Autodesk Fusion 360 part; units mm, degrees
(part 4 of 7)
  line L870 (66.9243, -68.9138) -> (66.9958, -68.9472)
  line L871 (66.9958, -68.9472) -> (67.1016, -68.8548)
  line L872 (67.1016, -68.8548) -> (67.2059, -68.7609)
  line L873 (67.2059, -68.7609) -> (67.3089, -68.6653)
  line L874 (67.3089, -68.6653) -> (67.2831, -68.5907)
  line L875 (67.2831, -68.5907) -> (67.256, -68.5172)
  line L876 (67.256, -68.5172) -> (67.2276, -68.4449)
  line L877 (67.2276, -68.4449) -> (67.1977, -68.3739)
  line L878 (67.1977, -68.3739) -> (67.1663, -68.3041)
  line L879 (67.1663, -68.3041) -> (67.1335, -68.2357)
  line L880 (67.1335, -68.2357) -> (67.099, -68.1688)
  line L881 (67.099, -68.1688) -> (67.0628, -68.1036)
  line L882 (67.0628, -68.1036) -> (67.0248, -68.04)
  line L883 (67.0248, -68.04) -> (66.9847, -67.9785)
  line L884 (66.9847, -67.9785) -> (66.942, -67.9195)
  line L885 (66.942, -67.9195) -> (66.8957, -67.8642)
  line L886 (66.8957, -67.8642) -> (66.5795, -67.5479)
  line L887 (66.5795, -67.5479) -> (66.7269, -67.3967)
  line L888 (66.7269, -67.3967) -> (66.8702, -67.2417)
  line L889 (66.8702, -67.2417) -> (67.0094, -67.0829)
  line L890 (67.0094, -67.0829) -> (67.1444, -66.9206)
  line L891 (67.1444, -66.9206) -> (67.492, -67.2019)
  line L892 (67.492, -67.2019) -> (67.5519, -67.2422)
  line L893 (67.5519, -67.2422) -> (67.615, -67.2785)
  line L894 (67.615, -67.2785) -> (67.6804, -67.3119)
  line L895 (67.6804, -67.3119) -> (67.7475, -67.3431)
  line L896 (67.7475, -67.3431) -> (67.8162, -67.3723)
  line L897 (67.8162, -67.3723) -> (67.8864, -67.3996)
  line L898 (67.8864, -67.3996) -> (67.9578, -67.4251)
  line L899 (67.9578, -67.4251) -> (68.0305, -67.449)
  line L900 (68.0305, -67.449) -> (68.1043, -67.4713)
  line L901 (68.1043, -67.4713) -> (68.1791, -67.492)
  line L902 (68.1791, -67.492) -> (68.255, -67.5113)
  line L903 (68.255, -67.5113) -> (68.3319, -67.5291)
  line L904 (68.3319, -67.5291) -> (68.4162, -67.4167)
  line L905 (68.4162, -67.4167) -> (68.4987, -67.3031)
  line L906 (68.4987, -67.3031) -> (68.5795, -67.1883)
  line L907 (68.5795, -67.1883) -> (68.5389, -67.1207)
  line L908 (68.5389, -67.1207) -> (68.4971, -67.0544)
  line L909 (68.4971, -67.0544) -> (68.4542, -66.9896)
  line L910 (68.4542, -66.9896) -> (68.4102, -66.9263)
  line L911 (68.4102, -66.9263) -> (68.365, -66.8646)
  line L912 (68.365, -66.8646) -> (68.3187, -66.8046)
  line L913 (68.3187, -66.8046) -> (68.271, -66.7463)
  line L914 (68.271, -66.7463) -> (68.2221, -66.6899)
  line L915 (68.2221, -66.6899) -> (68.1717, -66.6357)
  line L916 (68.1717, -66.6357) -> (68.1196, -66.5839)
  line L917 (68.1196, -66.5839) -> (68.0657, -66.535)
  line L918 (68.0657, -66.535) -> (68.0088, -66.4906)
  line L919 (68.0088, -66.4906) -> (67.6338, -66.2469)
  line L920 (67.6338, -66.2469) -> (67.7465, -66.0684)
  line L921 (67.7465, -66.0684) -> (67.8545, -65.8869)
  line L922 (67.8545, -65.8869) -> (67.9576, -65.7027)
  line L923 (67.9576, -65.7027) -> (68.0559, -65.5158)
  line L924 (68.0559, -65.5158) -> (68.4544, -65.7187)
  line L925 (68.4544, -65.7187) -> (68.5214, -65.7458)
  line L926 (68.5214, -65.7458) -> (68.5907, -65.7681)
  line L927 (68.5907, -65.7681) -> (68.6615, -65.7872)
  line L928 (68.6615, -65.7872) -> (68.7337, -65.8038)
  line L929 (68.7337, -65.8038) -> (68.807, -65.818)
  line L930 (68.807, -65.818) -> (68.8813, -65.8301)
  line L931 (68.8813, -65.8301) -> (68.9564, -65.8402)
  line L932 (68.9564, -65.8402) -> (69.0325, -65.8485)
  line L933 (69.0325, -65.8485) -> (69.1093, -65.855)
  line L934 (69.1093, -65.855) -> (69.1869, -65.8597)
  line L935 (69.1869, -65.8597) -> (69.2651, -65.8627)
  line L936 (69.2651, -65.8627) -> (69.344, -65.8642)
  line L937 (69.344, -65.8642) -> (69.4031, -65.7368)
  line L938 (69.4031, -65.7368) -> (69.4602, -65.6085)
  line L939 (69.4602, -65.6085) -> (69.5154, -65.4793)
  line L940 (69.5154, -65.4793) -> (69.4615, -65.4216)
  line L941 (69.4615, -65.4216) -> (69.4069, -65.3655)
  line L942 (69.4069, -65.3655) -> (69.3515, -65.3111)
  line L943 (69.3515, -65.3111) -> (69.2952, -65.2583)
  line L944 (69.2952, -65.2583) -> (69.2382, -65.2073)
  line L945 (69.2382, -65.2073) -> (69.1804, -65.1582)
  line L946 (69.1804, -65.1582) -> (69.1217, -65.1111)
  line L947 (69.1217, -65.1111) -> (69.0621, -65.0662)
  line L948 (69.0621, -65.0662) -> (69.0015, -65.0236)
  line L949 (69.0015, -65.0236) -> (68.9399, -64.9838)
  line L950 (68.9399, -64.9838) -> (68.8769, -64.9472)
  line L951 (68.8769, -64.9472) -> (68.812, -64.9156)
  line L952 (68.812, -64.9156) -> (68.3946, -64.7551)
  line L953 (68.3946, -64.7551) -> (68.4677, -64.5571)
  line L954 (68.4677, -64.5571) -> (68.5356, -64.3572)
  line L955 (68.5356, -64.3572) -> (68.5982, -64.1555)
  line L956 (68.5982, -64.1555) -> (68.6554, -63.9523)
  line L957 (68.6554, -63.9523) -> (69.0875, -64.0679)
  line L958 (69.0875, -64.0679) -> (69.1585, -64.0804)
  line L959 (69.1585, -64.0804) -> (69.231, -64.0878)
  line L960 (69.231, -64.0878) -> (69.3043, -64.0918)
  line L961 (69.3043, -64.0918) -> (69.3783, -64.093)
  line L962 (69.3783, -64.093) -> (69.4529, -64.0917)
  line L963 (69.4529, -64.0917) -> (69.5281, -64.0881)
  line L964 (69.5281, -64.0881) -> (69.6038, -64.0824)
  line L965 (69.6038, -64.0824) -> (69.6798, -64.0746)
  line L966 (69.6798, -64.0746) -> (69.7563, -64.065)
  line L967 (69.7563, -64.065) -> (69.8332, -64.0535)
  line L968 (69.8332, -64.0535) -> (69.9104, -64.0402)
  line L969 (69.9104, -64.0402) -> (69.9878, -64.0252)
  line L970 (69.9878, -64.0252) -> (70.0191, -63.8883)
  line L971 (70.0191, -63.8883) -> (70.0483, -63.7509)
  line L972 (70.0483, -63.7509) -> (70.0754, -63.6131)
  line L973 (70.0754, -63.6131) -> (70.0107, -63.5679)
  line L974 (70.0107, -63.5679) -> (69.9456, -63.5244)
  line L975 (69.9456, -63.5244) -> (69.8801, -63.4826)
  line L976 (69.8801, -63.4826) -> (69.8142, -63.4427)
  line L977 (69.8142, -63.4427) -> (69.7478, -63.4047)
  line L978 (69.7478, -63.4047) -> (69.681, -63.3687)
  line L979 (69.681, -63.3687) -> (69.6138, -63.3348)
  line L980 (69.6138, -63.3348) -> (69.5462, -63.3033)
  line L981 (69.5462, -63.3033) -> (69.4781, -63.2742)
  line L982 (69.4781, -63.2742) -> (69.4095, -63.2481)
  line L983 (69.4095, -63.2481) -> (69.3403, -63.2254)
  line L984 (69.3403, -63.2254) -> (69.2703, -63.2079)
  line L985 (69.2703, -63.2079) -> (68.8286, -63.1378)
  line L986 (68.8286, -63.1378) -> (68.8589, -62.9289)
  line L987 (68.8589, -62.9289) -> (68.8837, -62.7192)
  line L988 (68.8837, -62.7192) -> (68.903, -62.509)
  line L989 (68.903, -62.509) -> (68.9168, -62.2983)
  circle A0 centre (60.9176, -61.8819) radius 2
extrude "Extrude1''" add sketch "Sketch1 (3)" along normal blind 2 separate body makes body 5 in component "CT idler 2"
ref_plane "WorkPlane2" through (0, 0, 41.2) normal (0, 0, 1) x (1, 0, 0) in component "CT idler 2"
sketch "Sketch2 (2)" plane through (0, 0, 41.2) normal (0, 0, 1) x (1, 0, 0) in component "CT idler 2"
  line L0 (63.97, -62.3626) -> (64.2593, -62.4081)
  line L1 (64.2593, -62.4081) -> (64.3399, -62.409)
  line L2 (64.3399, -62.409) -> (64.422, -62.3998)
  line L3 (64.422, -62.3998) -> (64.5049, -62.3837)
  line L4 (64.5049, -62.3837) -> (64.5883, -62.3617)
  line L5 (64.5883, -62.3617) -> (64.6722, -62.3342)
  line L6 (64.6722, -62.3342) -> (64.7562, -62.3017)
  line L7 (64.7562, -62.3017) -> (64.8402, -62.2644)
  line L8 (64.8402, -62.2644) -> (64.9242, -62.2224)
  line L9 (64.9242, -62.2224) -> (65.0078, -62.1758)
  line L10 (65.0078, -62.1758) -> (65.091, -62.1248)
  line L11 (65.091, -62.1248) -> (65.1737, -62.0695)
  line L12 (65.1737, -62.0695) -> (65.2557, -62.0099)
  line L13 (65.2557, -62.0099) -> (65.2574, -61.9246)
  line L14 (65.2574, -61.9246) -> (65.2574, -61.8393)
  line L15 (65.2574, -61.8393) -> (65.2557, -61.754)
  line L16 (65.2557, -61.754) -> (65.1737, -61.6944)
  line L17 (65.1737, -61.6944) -> (65.091, -61.6391)
  line L18 (65.091, -61.6391) -> (65.0078, -61.5881)
  line L19 (65.0078, -61.5881) -> (64.9242, -61.5415)
  line L20 (64.9242, -61.5415) -> (64.8402, -61.4995)
  line L21 (64.8402, -61.4995) -> (64.7562, -61.4621)
  line L22 (64.7562, -61.4621) -> (64.6722, -61.4296)
  line L23 (64.6722, -61.4296) -> (64.5883, -61.4022)
  line L24 (64.5883, -61.4022) -> (64.5049, -61.3801)
  line L25 (64.5049, -61.3801) -> (64.422, -61.364)
  line L26 (64.422, -61.364) -> (64.3399, -61.3549)
  line L27 (64.3399, -61.3549) -> (64.2593, -61.3557)
  line L28 (64.2593, -61.3557) -> (63.97, -61.4013)
  line L29 (63.97, -61.4013) -> (63.9404, -61.2408)
  line L30 (63.9404, -61.2408) -> (63.9023, -61.0822)
  line L31 (63.9023, -61.0822) -> (63.856, -60.9257)
  line L32 (63.856, -60.9257) -> (63.8014, -60.772)
  line L33 (63.8014, -60.772) -> (64.0747, -60.6668)
  line L34 (64.0747, -60.6668) -> (64.145, -60.6272)
  line L35 (64.145, -60.6272) -> (64.2114, -60.5783)
  line L36 (64.2114, -60.5783) -> (64.2752, -60.5229)
  line L37 (64.2752, -60.5229) -> (64.3364, -60.4621)
  line L38 (64.3364, -60.4621) -> (64.3953, -60.3964)
  line L39 (64.3953, -60.3964) -> (64.4518, -60.3262)
  line L40 (64.4518, -60.3262) -> (64.5059, -60.2518)
  line L41 (64.5059, -60.2518) -> (64.5576, -60.1735)
  line L42 (64.5576, -60.1735) -> (64.6068, -60.0913)
  line L43 (64.6068, -60.0913) -> (64.6534, -60.0056)
  line L44 (64.6534, -60.0056) -> (64.6973, -59.9163)
  line L45 (64.6973, -59.9163) -> (64.7385, -59.8237)
  line L46 (64.7385, -59.8237) -> (64.6973, -59.749)
  line L47 (64.6973, -59.749) -> (64.6547, -59.6751)
  line L48 (64.6547, -59.6751) -> (64.6106, -59.6021)
  line L49 (64.6106, -59.6021) -> (64.5098, -59.5915)
  line L50 (64.5098, -59.5915) -> (64.4105, -59.5849)
  line L51 (64.4105, -59.5849) -> (64.3129, -59.5823)
  line L52 (64.3129, -59.5823) -> (64.2172, -59.5839)
  line L53 (64.2172, -59.5839) -> (64.1235, -59.5894)
  line L54 (64.1235, -59.5894) -> (64.032, -59.5991)
  line L55 (64.032, -59.5991) -> (63.943, -59.6129)
  line L56 (63.943, -59.6129) -> (63.8567, -59.6311)
  line L57 (63.8567, -59.6311) -> (63.7734, -59.6537)
  line L58 (63.7734, -59.6537) -> (63.6935, -59.6812)
  line L59 (63.6935, -59.6812) -> (63.6179, -59.7143)
  line L60 (63.6179, -59.7143) -> (63.5485, -59.7554)
  line L61 (63.5485, -59.7554) -> (63.3208, -59.9395)
  line L62 (63.3208, -59.9395) -> (63.2149, -59.8153)
  line L63 (63.2149, -59.8153) -> (63.1026, -59.697)
  line L64 (63.1026, -59.697) -> (62.9842, -59.5847)
  line L65 (62.9842, -59.5847) -> (62.8601, -59.4788)
  line L66 (62.8601, -59.4788) -> (63.0442, -59.251)
  line L67 (63.0442, -59.251) -> (63.0852, -59.1816)
  line L68 (63.0852, -59.1816) -> (63.1183, -59.106)
  line L69 (63.1183, -59.106) -> (63.1458, -59.0262)
  line L70 (63.1458, -59.0262) -> (63.1685, -58.9429)
  line L71 (63.1685, -58.9429) -> (63.1866, -58.8566)
  line L72 (63.1866, -58.8566) -> (63.2005, -58.7675)
  line L73 (63.2005, -58.7675) -> (63.2101, -58.6761)
  line L74 (63.2101, -58.6761) -> (63.2157, -58.5824)
  line L75 (63.2157, -58.5824) -> (63.2172, -58.4867)
  line L76 (63.2172, -58.4867) -> (63.2147, -58.3891)
  line L77 (63.2147, -58.3891) -> (63.2081, -58.2898)
  line L78 (63.2081, -58.2898) -> (63.1975, -58.189)
  line L79 (63.1975, -58.189) -> (63.1245, -58.1449)
  line L80 (63.1245, -58.1449) -> (63.0506, -58.1022)
  line L81 (63.0506, -58.1022) -> (62.9759, -58.061)
  line L82 (62.9759, -58.061) -> (62.8833, -58.1023)
  line L83 (62.8833, -58.1023) -> (62.794, -58.1462)
  line L84 (62.794, -58.1462) -> (62.7082, -58.1928)
  line L85 (62.7082, -58.1928) -> (62.6261, -58.242)
  line L86 (62.6261, -58.242) -> (62.5477, -58.2936)
  line L87 (62.5477, -58.2936) -> (62.4733, -58.3477)
  line L88 (62.4733, -58.3477) -> (62.4032, -58.4042)
  line L89 (62.4032, -58.4042) -> (62.3375, -58.4631)
  line L90 (62.3375, -58.4631) -> (62.2767, -58.5244)
  line L91 (62.2767, -58.5244) -> (62.2213, -58.5881)
  line L92 (62.2213, -58.5881) -> (62.1723, -58.6546)
  line L93 (62.1723, -58.6546) -> (62.1328, -58.7248)
  line L94 (62.1328, -58.7248) -> (62.0276, -58.9982)
  line L95 (62.0276, -58.9982) -> (61.8738, -58.9436)
  line L96 (61.8738, -58.9436) -> (61.7174, -58.8972)
  line L97 (61.7174, -58.8972) -> (61.5587, -58.8592)
  line L98 (61.5587, -58.8592) -> (61.3983, -58.8295)
  line L99 (61.3983, -58.8295) -> (61.4438, -58.5402)
  line L100 (61.4438, -58.5402) -> (61.4447, -58.4596)
  line L101 (61.4447, -58.4596) -> (61.4355, -58.3776)
  line L102 (61.4355, -58.3776) -> (61.4194, -58.2947)
  line L103 (61.4194, -58.2947) -> (61.3974, -58.2112)
  line L104 (61.3974, -58.2112) -> (61.3699, -58.1274)
  line L105 (61.3699, -58.1274) -> (61.3374, -58.0434)
  line L106 (61.3374, -58.0434) -> (61.3001, -57.9593)
  line L107 (61.3001, -57.9593) -> (61.258, -57.8754)
  line L108 (61.258, -57.8754) -> (61.2115, -57.7917)
  line L109 (61.2115, -57.7917) -> (61.1605, -57.7085)
  line L110 (61.1605, -57.7085) -> (61.1052, -57.6258)
  line L111 (61.1052, -57.6258) -> (61.0456, -57.5438)
  line L112 (61.0456, -57.5438) -> (60.9603, -57.5421)
  line L113 (60.9603, -57.5421) -> (60.875, -57.5421)
  line L114 (60.875, -57.5421) -> (60.7897, -57.5438)
  line L115 (60.7897, -57.5438) -> (60.7301, -57.6258)
  line L116 (60.7301, -57.6258) -> (60.6747, -57.7085)
  line L117 (60.6747, -57.7085) -> (60.6238, -57.7917)
  line L118 (60.6238, -57.7917) -> (60.5772, -57.8754)
  line L119 (60.5772, -57.8754) -> (60.5352, -57.9593)
  line L120 (60.5352, -57.9593) -> (60.4978, -58.0434)
  line L121 (60.4978, -58.0434) -> (60.4653, -58.1274)
  line L122 (60.4653, -58.1274) -> (60.4379, -58.2112)
  line L123 (60.4379, -58.2112) -> (60.4158, -58.2947)
  line L124 (60.4158, -58.2947) -> (60.3997, -58.3776)
  line L125 (60.3997, -58.3776) -> (60.3906, -58.4596)
  line L126 (60.3906, -58.4596) -> (60.3914, -58.5402)
  line L127 (60.3914, -58.5402) -> (60.437, -58.8295)
  line L128 (60.437, -58.8295) -> (60.2765, -58.8592)
  line L129 (60.2765, -58.8592) -> (60.1179, -58.8972)
  line L130 (60.1179, -58.8972) -> (59.9614, -58.9436)
  line L131 (59.9614, -58.9436) -> (59.8077, -58.9982)
  line L132 (59.8077, -58.9982) -> (59.7025, -58.7248)
  line L133 (59.7025, -58.7248) -> (59.6629, -58.6546)
  line L134 (59.6629, -58.6546) -> (59.614, -58.5881)
  line L135 (59.614, -58.5881) -> (59.5586, -58.5244)
  line L136 (59.5586, -58.5244) -> (59.4978, -58.4631)
  line L137 (59.4978, -58.4631) -> (59.4321, -58.4042)
  line L138 (59.4321, -58.4042) -> (59.3619, -58.3477)
  line L139 (59.3619, -58.3477) -> (59.2875, -58.2936)
  line L140 (59.2875, -58.2936) -> (59.2092, -58.242)
  line L141 (59.2092, -58.242) -> (59.127, -58.1928)
  line L142 (59.127, -58.1928) -> (59.0412, -58.1462)
  line L143 (59.0412, -58.1462) -> (58.952, -58.1023)
  line L144 (58.952, -58.1023) -> (58.8594, -58.061)
  line L145 (58.8594, -58.061) -> (58.7847, -58.1022)
  line L146 (58.7847, -58.1022) -> (58.7108, -58.1449)
  line L147 (58.7108, -58.1449) -> (58.6378, -58.189)
  line L148 (58.6378, -58.189) -> (58.6272, -58.2898)
  line L149 (58.6272, -58.2898) -> (58.6206, -58.3891)
  line L150 (58.6206, -58.3891) -> (58.618, -58.4867)
  line L151 (58.618, -58.4867) -> (58.6195, -58.5824)
  line L152 (58.6195, -58.5824) -> (58.6251, -58.6761)
  line L153 (58.6251, -58.6761) -> (58.6348, -58.7675)
  line L154 (58.6348, -58.7675) -> (58.6486, -58.8566)
  line L155 (58.6486, -58.8566) -> (58.6668, -58.9429)
  line L156 (58.6668, -58.9429) -> (58.6894, -59.0262)
  line L157 (58.6894, -59.0262) -> (58.7169, -59.106)
  line L158 (58.7169, -59.106) -> (58.75, -59.1816)
  line L159 (58.75, -59.1816) -> (58.7911, -59.251)
  line L160 (58.7911, -59.251) -> (58.9752, -59.4788)
  line L161 (58.9752, -59.4788) -> (58.851, -59.5847)
  line L162 (58.851, -59.5847) -> (58.7327, -59.697)
  line L163 (58.7327, -59.697) -> (58.6204, -59.8153)
  line L164 (58.6204, -59.8153) -> (58.5145, -59.9395)
  line L165 (58.5145, -59.9395) -> (58.2867, -59.7554)
  line L166 (58.2867, -59.7554) -> (58.2173, -59.7143)
  line L167 (58.2173, -59.7143) -> (58.1417, -59.6812)
  line L168 (58.1417, -59.6812) -> (58.0619, -59.6537)
  line L169 (58.0619, -59.6537) -> (57.9786, -59.6311)
  line L170 (57.9786, -59.6311) -> (57.8923, -59.6129)
  line L171 (57.8923, -59.6129) -> (57.8032, -59.5991)
  line L172 (57.8032, -59.5991) -> (57.7118, -59.5894)
  line L173 (57.7118, -59.5894) -> (57.6181, -59.5839)
  line L174 (57.6181, -59.5839) -> (57.5224, -59.5823)
  line L175 (57.5224, -59.5823) -> (57.4248, -59.5849)
  line L176 (57.4248, -59.5849) -> (57.3255, -59.5915)
  line L177 (57.3255, -59.5915) -> (57.2247, -59.6021)
  line L178 (57.2247, -59.6021) -> (57.1806, -59.6751)
  line L179 (57.1806, -59.6751) -> (57.1379, -59.749)
  line L180 (57.1379, -59.749) -> (57.0967, -59.8237)
  line L181 (57.0967, -59.8237) -> (57.138, -59.9163)
  line L182 (57.138, -59.9163) -> (57.1819, -60.0056)
  line L183 (57.1819, -60.0056) -> (57.2285, -60.0913)
  line L184 (57.2285, -60.0913) -> (57.2777, -60.1735)
  line L185 (57.2777, -60.1735) -> (57.3293, -60.2518)
  line L186 (57.3293, -60.2518) -> (57.3834, -60.3262)
  line L187 (57.3834, -60.3262) -> (57.4399, -60.3964)
  line L188 (57.4399, -60.3964) -> (57.4988, -60.4621)
  line L189 (57.4988, -60.4621) -> (57.5601, -60.5229)
  line L190 (57.5601, -60.5229) -> (57.6238, -60.5783)
  line L191 (57.6238, -60.5783) -> (57.6903, -60.6272)
  line L192 (57.6903, -60.6272) -> (57.7605, -60.6668)
  line L193 (57.7605, -60.6668) -> (58.0339, -60.772)
  line L194 (58.0339, -60.772) -> (57.9793, -60.9257)
  line L195 (57.9793, -60.9257) -> (57.9329, -61.0822)
  line L196 (57.9329, -61.0822) -> (57.8949, -61.2408)
  line L197 (57.8949, -61.2408) -> (57.8652, -61.4013)
  line L198 (57.8652, -61.4013) -> (57.5759, -61.3557)
  line L199 (57.5759, -61.3557) -> (57.4953, -61.3549)
  line L200 (57.4953, -61.3549) -> (57.4133, -61.364)
  line L201 (57.4133, -61.364) -> (57.3304, -61.3801)
  line L202 (57.3304, -61.3801) -> (57.2469, -61.4022)
  line L203 (57.2469, -61.4022) -> (57.1631, -61.4296)
  line L204 (57.1631, -61.4296) -> (57.0791, -61.4621)
  line L205 (57.0791, -61.4621) -> (56.995, -61.4995)
  line L206 (56.995, -61.4995) -> (56.9111, -61.5415)
  line L207 (56.9111, -61.5415) -> (56.8274, -61.5881)
  line L208 (56.8274, -61.5881) -> (56.7442, -61.6391)
  line L209 (56.7442, -61.6391) -> (56.6615, -61.6944)
  line L210 (56.6615, -61.6944) -> (56.5795, -61.754)
  line L211 (56.5795, -61.754) -> (56.5778, -61.8393)
  line L212 (56.5778, -61.8393) -> (56.5778, -61.9246)
  line L213 (56.5778, -61.9246) -> (56.5795, -62.0099)
  line L214 (56.5795, -62.0099) -> (56.6615, -62.0695)
  line L215 (56.6615, -62.0695) -> (56.7442, -62.1248)
  line L216 (56.7442, -62.1248) -> (56.8274, -62.1758)
  line L217 (56.8274, -62.1758) -> (56.9111, -62.2224)
  line L218 (56.9111, -62.2224) -> (56.995, -62.2644)
  line L219 (56.995, -62.2644) -> (57.0791, -62.3017)
  line L220 (57.0791, -62.3017) -> (57.1631, -62.3342)
  line L221 (57.1631, -62.3342) -> (57.2469, -62.3617)
  line L222 (57.2469, -62.3617) -> (57.3304, -62.3837)
  line L223 (57.3304, -62.3837) -> (57.4133, -62.3998)
  line L224 (57.4133, -62.3998) -> (57.4953, -62.409)
  line L225 (57.4953, -62.409) -> (57.5759, -62.4081)
  line L226 (57.5759, -62.4081) -> (57.8652, -62.3626)
  line L227 (57.8652, -62.3626) -> (57.8949, -62.523)
  line L228 (57.8949, -62.523) -> (57.9329, -62.6817)
  line L229 (57.9329, -62.6817) -> (57.9793, -62.8381)
  line L230 (57.9793, -62.8381) -> (58.0339, -62.9919)
  line L231 (58.0339, -62.9919) -> (57.7605, -63.0971)
  line L232 (57.7605, -63.0971) -> (57.6903, -63.1366)
  line L233 (57.6903, -63.1366) -> (57.6238, -63.1856)
  line L234 (57.6238, -63.1856) -> (57.5601, -63.241)
  line L235 (57.5601, -63.241) -> (57.4988, -63.3018)
  line L236 (57.4988, -63.3018) -> (57.4399, -63.3675)
  line L237 (57.4399, -63.3675) -> (57.3834, -63.4377)
  line L238 (57.3834, -63.4377) -> (57.3293, -63.512)
  line L239 (57.3293, -63.512) -> (57.2777, -63.5904)
  line L240 (57.2777, -63.5904) -> (57.2285, -63.6725)
  line L241 (57.2285, -63.6725) -> (57.1819, -63.7583)
  line L242 (57.1819, -63.7583) -> (57.138, -63.8476)
  line L243 (57.138, -63.8476) -> (57.0967, -63.9402)
  line L244 (57.0967, -63.9402) -> (57.1379, -64.0149)
  line L245 (57.1379, -64.0149) -> (57.1806, -64.0888)
  line L246 (57.1806, -64.0888) -> (57.2247, -64.1618)
  line L247 (57.2247, -64.1618) -> (57.3255, -64.1724)
  line L248 (57.3255, -64.1724) -> (57.4248, -64.179)
  line L249 (57.4248, -64.179) -> (57.5224, -64.1815)
  line L250 (57.5224, -64.1815) -> (57.6181, -64.18)
  line L251 (57.6181, -64.18) -> (57.7118, -64.1744)
  line L252 (57.7118, -64.1744) -> (57.8032, -64.1648)
  line L253 (57.8032, -64.1648) -> (57.8923, -64.1509)
  line L254 (57.8923, -64.1509) -> (57.9786, -64.1328)
  line L255 (57.9786, -64.1328) -> (58.0619, -64.1101)
  line L256 (58.0619, -64.1101) -> (58.1417, -64.0826)
  line L257 (58.1417, -64.0826) -> (58.2173, -64.0495)
  line L258 (58.2173, -64.0495) -> (58.2867, -64.0085)
  line L259 (58.2867, -64.0085) -> (58.5145, -63.8244)
  line L260 (58.5145, -63.8244) -> (58.6204, -63.9485)
  line L261 (58.6204, -63.9485) -> (58.7327, -64.0669)
  line L262 (58.7327, -64.0669) -> (58.851, -64.1792)
  line L263 (58.851, -64.1792) -> (58.9752, -64.2851)
  line L264 (58.9752, -64.2851) -> (58.7911, -64.5128)
  line L265 (58.7911, -64.5128) -> (58.75, -64.5822)
  line L266 (58.75, -64.5822) -> (58.7169, -64.6578)
  line L267 (58.7169, -64.6578) -> (58.6894, -64.7377)
  line L268 (58.6894, -64.7377) -> (58.6668, -64.821)
  line L269 (58.6668, -64.821) -> (58.6486, -64.9073)
  line L270 (58.6486, -64.9073) -> (58.6348, -64.9963)
  line L271 (58.6348, -64.9963) -> (58.6251, -65.0878)
  line L272 (58.6251, -65.0878) -> (58.6195, -65.1815)
  line L273 (58.6195, -65.1815) -> (58.618, -65.2772)
  line L274 (58.618, -65.2772) -> (58.6206, -65.3748)
  line L275 (58.6206, -65.3748) -> (58.6272, -65.4741)
  line L276 (58.6272, -65.4741) -> (58.6378, -65.5749)
  line L277 (58.6378, -65.5749) -> (58.7108, -65.619)
  line L278 (58.7108, -65.619) -> (58.7847, -65.6616)
  line L279 (58.7847, -65.6616) -> (58.8594, -65.7028)
  line L280 (58.8594, -65.7028) -> (58.952, -65.6616)
  line L281 (58.952, -65.6616) -> (59.0412, -65.6177)
  line L282 (59.0412, -65.6177) -> (59.127, -65.5711)
  line L283 (59.127, -65.5711) -> (59.2092, -65.5219)
  line L284 (59.2092, -65.5219) -> (59.2875, -65.4702)
  line L285 (59.2875, -65.4702) -> (59.3619, -65.4161)
  line L286 (59.3619, -65.4161) -> (59.4321, -65.3596)
  line L287 (59.4321, -65.3596) -> (59.4978, -65.3007)
  line L288 (59.4978, -65.3007) -> (59.5586, -65.2395)
  line L289 (59.5586, -65.2395) -> (59.614, -65.1757)
  line L290 (59.614, -65.1757) -> (59.6629, -65.1093)
  line L291 (59.6629, -65.1093) -> (59.7025, -65.039)
  line L292 (59.7025, -65.039) -> (59.8077, -64.7657)
  line L293 (59.8077, -64.7657) -> (59.9614, -64.8203)
  line L294 (59.9614, -64.8203) -> (60.1179, -64.8666)
  line L295 (60.1179, -64.8666) -> (60.2765, -64.9047)
  line L296 (60.2765, -64.9047) -> (60.437, -64.9343)
  line L297 (60.437, -64.9343) -> (60.3914, -65.2236)
  line L298 (60.3914, -65.2236) -> (60.3906, -65.3042)
  line L299 (60.3906, -65.3042) -> (60.3997, -65.3863)
  line L300 (60.3997, -65.3863) -> (60.4158, -65.4692)
  line L301 (60.4158, -65.4692) -> (60.4379, -65.5526)
  line L302 (60.4379, -65.5526) -> (60.4653, -65.6365)
  line L303 (60.4653, -65.6365) -> (60.4978, -65.7205)
  line L304 (60.4978, -65.7205) -> (60.5352, -65.8045)
  line L305 (60.5352, -65.8045) -> (60.5772, -65.8885)
  line L306 (60.5772, -65.8885) -> (60.6238, -65.9721)
  line L307 (60.6238, -65.9721) -> (60.6747, -66.0554)
  line L308 (60.6747, -66.0554) -> (60.7301, -66.138)
  line L309 (60.7301, -66.138) -> (60.7897, -66.22)
  line L310 (60.7897, -66.22) -> (60.875, -66.2217)
  line L311 (60.875, -66.2217) -> (60.9603, -66.2217)
  line L312 (60.9603, -66.2217) -> (61.0456, -66.22)
  line L313 (61.0456, -66.22) -> (61.1052, -66.138)
  line L314 (61.1052, -66.138) -> (61.1605, -66.0554)
  line L315 (61.1605, -66.0554) -> (61.2115, -65.9721)
  line L316 (61.2115, -65.9721) -> (61.258, -65.8885)
  line L317 (61.258, -65.8885) -> (61.3001, -65.8045)
  line L318 (61.3001, -65.8045) -> (61.3374, -65.7205)
  line L319 (61.3374, -65.7205) -> (61.3699, -65.6365)
  line L320 (61.3699, -65.6365) -> (61.3974, -65.5526)
  line L321 (61.3974, -65.5526) -> (61.4194, -65.4692)
  line L322 (61.4194, -65.4692) -> (61.4355, -65.3863)
  line L323 (61.4355, -65.3863) -> (61.4447, -65.3042)
  line L324 (61.4447, -65.3042) -> (61.4438, -65.2236)
  line L325 (61.4438, -65.2236) -> (61.3983, -64.9343)
  line L326 (61.3983, -64.9343) -> (61.5587, -64.9047)
  line L327 (61.5587, -64.9047) -> (61.7174, -64.8666)
  line L328 (61.7174, -64.8666) -> (61.8738, -64.8203)
  line L329 (61.8738, -64.8203) -> (62.0276, -64.7657)
  line L330 (62.0276, -64.7657) -> (62.1328, -65.039)
  line L331 (62.1328, -65.039) -> (62.1723, -65.1093)
  line L332 (62.1723, -65.1093) -> (62.2213, -65.1757)
  line L333 (62.2213, -65.1757) -> (62.2767, -65.2395)
  line L334 (62.2767, -65.2395) -> (62.3375, -65.3007)
  line L335 (62.3375, -65.3007) -> (62.4032, -65.3596)
  line L336 (62.4032, -65.3596) -> (62.4733, -65.4161)
  line L337 (62.4733, -65.4161) -> (62.5477, -65.4702)
  line L338 (62.5477, -65.4702) -> (62.6261, -65.5219)
  line L339 (62.6261, -65.5219) -> (62.7082, -65.5711)
  line L340 (62.7082, -65.5711) -> (62.794, -65.6177)
  line L341 (62.794, -65.6177) -> (62.8833, -65.6616)
  line L342 (62.8833, -65.6616) -> (62.9759, -65.7028)
  line L343 (62.9759, -65.7028) -> (63.0506, -65.6616)
  line L344 (63.0506, -65.6616) -> (63.1245, -65.619)
  line L345 (63.1245, -65.619) -> (63.1975, -65.5749)
  line L346 (63.1975, -65.5749) -> (63.2081, -65.4741)
  line L347 (63.2081, -65.4741) -> (63.2147, -65.3748)
  line L348 (63.2147, -65.3748) -> (63.2172, -65.2772)
  line L349 (63.2172, -65.2772) -> (63.2157, -65.1815)
  line L350 (63.2157, -65.1815) -> (63.2101, -65.0878)
  line L351 (63.2101, -65.0878) -> (63.2005, -64.9963)
  line L352 (63.2005, -64.9963) -> (63.1866, -64.9073)
  line L353 (63.1866, -64.9073) -> (63.1685, -64.821)
  line L354 (63.1685, -64.821) -> (63.1458, -64.7377)
  line L355 (63.1458, -64.7377) -> (63.1183, -64.6578)
  line L356 (63.1183, -64.6578) -> (63.0852, -64.5822)
  line L357 (63.0852, -64.5822) -> (63.0442, -64.5128)
  line L358 (63.0442, -64.5128) -> (62.8601, -64.2851)
  line L359 (62.8601, -64.2851) -> (62.9842, -64.1792)
  line L360 (62.9842, -64.1792) -> (63.1026, -64.0669)
  line L361 (63.1026, -64.0669) -> (63.2149, -63.9485)
  line L362 (63.2149, -63.9485) -> (63.3208, -63.8244)
  line L363 (63.3208, -63.8244) -> (63.5485, -64.0085)
  line L364 (63.5485, -64.0085) -> (63.6179, -64.0495)
  line L365 (63.6179, -64.0495) -> (63.6935, -64.0826)
  line L366 (63.6935, -64.0826) -> (63.7734, -64.1101)
  line L367 (63.7734, -64.1101) -> (63.8567, -64.1328)
  line L368 (63.8567, -64.1328) -> (63.943, -64.1509)
  line L369 (63.943, -64.1509) -> (64.032, -64.1648)
  line L370 (64.032, -64.1648) -> (64.1235, -64.1744)
  line L371 (64.1235, -64.1744) -> (64.2172, -64.18)
  line L372 (64.2172, -64.18) -> (64.3129, -64.1815)
  line L373 (64.3129, -64.1815) -> (64.4105, -64.179)
  line L374 (64.4105, -64.179) -> (64.5098, -64.1724)
  line L375 (64.5098, -64.1724) -> (64.6106, -64.1618)
  line L376 (64.6106, -64.1618) -> (64.6547, -64.0888)
  line L377 (64.6547, -64.0888) -> (64.6973, -64.0149)
  line L378 (64.6973, -64.0149) -> (64.7385, -63.9402)
  line L379 (64.7385, -63.9402) -> (64.6973, -63.8476)
  line L380 (64.6973, -63.8476) -> (64.6534, -63.7583)
  line L381 (64.6534, -63.7583) -> (64.6068, -63.6725)
  line L382 (64.6068, -63.6725) -> (64.5576, -63.5904)
  line L383 (64.5576, -63.5904) -> (64.5059, -63.512)
  line L384 (64.5059, -63.512) -> (64.4518, -63.4377)
  line L385 (64.4518, -63.4377) -> (64.3953, -63.3675)
  line L386 (64.3953, -63.3675) -> (64.3364, -63.3018)
  line L387 (64.3364, -63.3018) -> (64.2752, -63.241)
  line L388 (64.2752, -63.241) -> (64.2114, -63.1856)
  line L389 (64.2114, -63.1856) -> (64.145, -63.1366)
  line L390 (64.145, -63.1366) -> (64.0747, -63.0971)
  line L391 (64.0747, -63.0971) -> (63.8014, -62.9919)
  line L392 (63.8014, -62.9919) -> (63.856, -62.8381)
  line L393 (63.856, -62.8381) -> (63.9023, -62.6817)
  line L394 (63.9023, -62.6817) -> (63.9404, -62.523)
  line L395 (63.9404, -62.523) -> (63.97, -62.3626)
  circle A0 centre (60.9176, -61.8819) radius 2
extrude "Extrude2'" add sketch "Sketch2 (2)" along normal blind 2 separate body makes body 6 in component "CT idler 2"
combine "Combine1'" operation add target body 5 tool bodies 6 makes body 7 at (59.5668, -59.5423, 41.2) in component "CT idler 2"
ref_plane "WorkPlane1" through (0, 0, 41.2) normal (0, 0, 1) x (1, 0, 0) in component "CT idler 3"
sketch "Sketch1 (4)" plane through (0, 0, 41.2) normal (0, 0, 1) x (1, 0, 0) in component "CT idler 3"
  line L0 (72.6858, -50.2752) -> (73.1324, -50.2984)
  line L1 (73.1324, -50.2984) -> (73.2045, -50.2959)
  line L2 (73.2045, -50.2959) -> (73.2769, -50.2881)
  line L3 (73.2769, -50.2881) -> (73.3494, -50.2768)
  line L4 (73.3494, -50.2768) -> (73.4221, -50.2625)
  line L5 (73.4221, -50.2625) -> (73.4948, -50.2457)
  line L6 (73.4948, -50.2457) -> (73.5676, -50.2266)
  line L7 (73.5676, -50.2266) -> (73.6404, -50.2052)
  line L8 (73.6404, -50.2052) -> (73.7132, -50.1819)
  line L9 (73.7132, -50.1819) -> (73.786, -50.1565)
  line L10 (73.786, -50.1565) -> (73.8588, -50.1293)
  line L11 (73.8588, -50.1293) -> (73.9315, -50.1003)
  line L12 (73.9315, -50.1003) -> (74.0042, -50.0695)
  line L13 (74.0042, -50.0695) -> (74.0063, -49.929)
  line L14 (74.0063, -49.929) -> (74.0063, -49.7886)
  line L15 (74.0063, -49.7886) -> (74.0042, -49.6482)
  line L16 (74.0042, -49.6482) -> (73.9315, -49.6174)
  line L17 (73.9315, -49.6174) -> (73.8588, -49.5884)
  line L18 (73.8588, -49.5884) -> (73.786, -49.5611)
  line L19 (73.786, -49.5611) -> (73.7132, -49.5358)
  line L20 (73.7132, -49.5358) -> (73.6404, -49.5124)
  line L21 (73.6404, -49.5124) -> (73.5676, -49.4911)
  line L22 (73.5676, -49.4911) -> (73.4948, -49.472)
  line L23 (73.4948, -49.472) -> (73.4221, -49.4551)
  line L24 (73.4221, -49.4551) -> (73.3494, -49.4409)
  line L25 (73.3494, -49.4409) -> (73.2769, -49.4296)
  line L26 (73.2769, -49.4296) -> (73.2045, -49.4218)
  line L27 (73.2045, -49.4218) -> (73.1324, -49.4192)
  line L28 (73.1324, -49.4192) -> (72.6858, -49.4425)
  line L29 (72.6858, -49.4425) -> (72.672, -49.2318)
  line L30 (72.672, -49.2318) -> (72.6527, -49.0216)
  line L31 (72.6527, -49.0216) -> (72.6279, -48.8119)
  line L32 (72.6279, -48.8119) -> (72.5975, -48.603)
  line L33 (72.5975, -48.603) -> (73.0392, -48.5328)
  line L34 (73.0392, -48.5328) -> (73.1092, -48.5154)
  line L35 (73.1092, -48.5154) -> (73.1784, -48.4927)
  line L36 (73.1784, -48.4927) -> (73.247, -48.4665)
  line L37 (73.247, -48.4665) -> (73.3151, -48.4375)
  line L38 (73.3151, -48.4375) -> (73.3828, -48.4059)
  line L39 (73.3828, -48.4059) -> (73.45, -48.3721)
  line L40 (73.45, -48.3721) -> (73.5168, -48.3361)
  line L41 (73.5168, -48.3361) -> (73.5831, -48.2981)
  line L42 (73.5831, -48.2981) -> (73.6491, -48.2581)
  line L43 (73.6491, -48.2581) -> (73.7146, -48.2164)
  line L44 (73.7146, -48.2164) -> (73.7797, -48.1728)
  line L45 (73.7797, -48.1728) -> (73.8444, -48.1276)
  line L46 (73.8444, -48.1276) -> (73.8173, -47.9898)
  line L47 (73.8173, -47.9898) -> (73.7881, -47.8525)
  line L48 (73.7881, -47.8525) -> (73.7568, -47.7156)
  line L49 (73.7568, -47.7156) -> (73.6793, -47.7005)
  line L50 (73.6793, -47.7005) -> (73.6021, -47.6873)
  line L51 (73.6021, -47.6873) -> (73.5253, -47.6758)
  line L52 (73.5253, -47.6758) -> (73.4488, -47.6661)
  line L53 (73.4488, -47.6661) -> (73.3727, -47.6584)
  line L54 (73.3727, -47.6584) -> (73.2971, -47.6527)
  line L55 (73.2971, -47.6527) -> (73.2219, -47.6491)
  line L56 (73.2219, -47.6491) -> (73.1473, -47.6478)
  line L57 (73.1473, -47.6478) -> (73.0732, -47.6489)
  line L58 (73.0732, -47.6489) -> (72.9999, -47.6529)
  line L59 (72.9999, -47.6529) -> (72.9275, -47.6603)
  line L60 (72.9275, -47.6603) -> (72.8564, -47.6729)
  line L61 (72.8564, -47.6729) -> (72.4244, -47.7885)
  line L62 (72.4244, -47.7885) -> (72.3671, -47.5852)
  line L63 (72.3671, -47.5852) -> (72.3045, -47.3836)
  line L64 (72.3045, -47.3836) -> (72.2367, -47.1837)
  line L65 (72.2367, -47.1837) -> (72.1635, -46.9856)
  line L66 (72.1635, -46.9856) -> (72.581, -46.8252)
  line L67 (72.581, -46.8252) -> (72.6459, -46.7936)
  line L68 (72.6459, -46.7936) -> (72.7088, -46.757)
  line L69 (72.7088, -46.757) -> (72.7705, -46.7171)
  line L70 (72.7705, -46.7171) -> (72.8311, -46.6746)
  line L71 (72.8311, -46.6746) -> (72.8907, -46.6296)
  line L72 (72.8907, -46.6296) -> (72.9494, -46.5825)
  line L73 (72.9494, -46.5825) -> (73.0072, -46.5334)
  line L74 (73.0072, -46.5334) -> (73.0642, -46.4825)
  line L75 (73.0642, -46.4825) -> (73.1204, -46.4297)
  line L76 (73.1204, -46.4297) -> (73.1758, -46.3752)
  line L77 (73.1758, -46.3752) -> (73.2305, -46.3191)
  line L78 (73.2305, -46.3191) -> (73.2843, -46.2614)
  line L79 (73.2843, -46.2614) -> (73.2291, -46.1323)
  line L80 (73.2291, -46.1323) -> (73.172, -46.004)
  line L81 (73.172, -46.004) -> (73.113, -45.8766)
  line L82 (73.113, -45.8766) -> (73.0341, -45.878)
  line L83 (73.0341, -45.878) -> (72.9558, -45.8811)
  line L84 (72.9558, -45.8811) -> (72.8783, -45.8858)
  line L85 (72.8783, -45.8858) -> (72.8014, -45.8923)
  line L86 (72.8014, -45.8923) -> (72.7254, -45.9005)
  line L87 (72.7254, -45.9005) -> (72.6502, -45.9107)
  line L88 (72.6502, -45.9107) -> (72.5759, -45.9228)
  line L89 (72.5759, -45.9228) -> (72.5027, -45.937)
  line L90 (72.5027, -45.937) -> (72.4305, -45.9535)
  line L91 (72.4305, -45.9535) -> (72.3596, -45.9727)
  line L92 (72.3596, -45.9727) -> (72.2903, -45.995)
  line L93 (72.2903, -45.995) -> (72.2234, -46.022)
  line L94 (72.2234, -46.022) -> (71.8248, -46.2249)
  line L95 (71.8248, -46.2249) -> (71.7266, -46.038)
  line L96 (71.7266, -46.038) -> (71.6234, -45.8538)
  line L97 (71.6234, -45.8538) -> (71.5155, -45.6724)
  line L98 (71.5155, -45.6724) -> (71.4028, -45.4939)
  line L99 (71.4028, -45.4939) -> (71.7778, -45.2502)
  line L100 (71.7778, -45.2502) -> (71.8346, -45.2057)
  line L101 (71.8346, -45.2057) -> (71.8886, -45.1568)
  line L102 (71.8886, -45.1568) -> (71.9406, -45.105)
  line L103 (71.9406, -45.105) -> (71.991, -45.0508)
  line L104 (71.991, -45.0508) -> (72.04, -44.9945)
  line L105 (72.04, -44.9945) -> (72.0876, -44.9362)
  line L106 (72.0876, -44.9362) -> (72.134, -44.8762)
  line L107 (72.134, -44.8762) -> (72.1792, -44.8144)
  line L108 (72.1792, -44.8144) -> (72.2232, -44.7511)
  line L109 (72.2232, -44.7511) -> (72.266, -44.6863)
  line L110 (72.266, -44.6863) -> (72.3078, -44.6201)
  line L111 (72.3078, -44.6201) -> (72.3485, -44.5525)
  line L112 (72.3485, -44.5525) -> (72.2677, -44.4376)
  line L113 (72.2677, -44.4376) -> (72.1851, -44.324)
  line L114 (72.1851, -44.324) -> (72.1009, -44.2117)
  line L115 (72.1009, -44.2117) -> (72.024, -44.2295)
  line L116 (72.024, -44.2295) -> (71.9481, -44.2487)
  line L117 (71.9481, -44.2487) -> (71.8732, -44.2695)
  line L118 (71.8732, -44.2695) -> (71.7994, -44.2918)
  line L119 (71.7994, -44.2918) -> (71.7268, -44.3157)
  line L120 (71.7268, -44.3157) -> (71.6553, -44.3412)
  line L121 (71.6553, -44.3412) -> (71.5852, -44.3685)
  line L122 (71.5852, -44.3685) -> (71.5165, -44.3976)
  line L123 (71.5165, -44.3976) -> (71.4493, -44.4288)
  line L124 (71.4493, -44.4288) -> (71.384, -44.4623)
  line L125 (71.384, -44.4623) -> (71.3208, -44.4985)
  line L126 (71.3208, -44.4985) -> (71.261, -44.5389)
  line L127 (71.261, -44.5389) -> (70.9133, -44.8202)
  line L128 (70.9133, -44.8202) -> (70.7784, -44.6578)
  line L129 (70.7784, -44.6578) -> (70.6392, -44.4991)
  line L130 (70.6392, -44.4991) -> (70.4959, -44.3441)
  line L131 (70.4959, -44.3441) -> (70.3485, -44.1929)
  line L132 (70.3485, -44.1929) -> (70.6646, -43.8765)
  line L133 (70.6646, -43.8765) -> (70.711, -43.8212)
  line L134 (70.711, -43.8212) -> (70.7536, -43.7622)
  line L135 (70.7536, -43.7622) -> (70.7937, -43.7007)
  line L136 (70.7937, -43.7007) -> (70.8318, -43.6372)
  line L137 (70.8318, -43.6372) -> (70.8679, -43.5719)
  line L138 (70.8679, -43.5719) -> (70.9024, -43.505)
  line L139 (70.9024, -43.505) -> (70.9353, -43.4366)
  line L140 (70.9353, -43.4366) -> (70.9666, -43.3669)
  line L141 (70.9666, -43.3669) -> (70.9965, -43.2958)
  line L142 (70.9965, -43.2958) -> (71.025, -43.2235)
  line L143 (71.025, -43.2235) -> (71.0521, -43.15)
  line L144 (71.0521, -43.15) -> (71.0778, -43.0754)
  line L145 (71.0778, -43.0754) -> (70.9749, -42.9799)
  line L146 (70.9749, -42.9799) -> (70.8705, -42.8859)
  line L147 (70.8705, -42.8859) -> (70.7648, -42.7936)
  line L148 (70.7648, -42.7936) -> (70.6933, -42.8269)
  line L149 (70.6933, -42.8269) -> (70.623, -42.8616)
  line L150 (70.623, -42.8616) -> (70.5541, -42.8974)
  line L151 (70.5541, -42.8974) -> (70.4865, -42.9346)
  line L152 (70.4865, -42.9346) -> (70.4204, -42.9731)
  line L153 (70.4204, -42.9731) -> (70.3559, -43.0129)
  line L154 (70.3559, -43.0129) -> (70.2929, -43.0542)
  line L155 (70.2929, -43.0542) -> (70.2318, -43.097)
  line L156 (70.2318, -43.097) -> (70.1726, -43.1414)
  line L157 (70.1726, -43.1414) -> (70.1156, -43.1878)
  line L158 (70.1156, -43.1878) -> (70.0614, -43.2363)
  line L159 (70.0614, -43.2363) -> (70.0112, -43.2882)
  line L160 (70.0112, -43.2882) -> (69.7297, -43.6357)
  line L161 (69.7297, -43.6357) -> (69.5639, -43.5049)
  line L162 (69.5639, -43.5049) -> (69.3947, -43.3786)
  line L163 (69.3947, -43.3786) -> (69.2223, -43.2568)
  line L164 (69.2223, -43.2568) -> (69.0467, -43.1395)
  line L165 (69.0467, -43.1395) -> (69.2902, -42.7644)
  line L166 (69.2902, -42.7644) -> (69.3241, -42.7006)
  line L167 (69.3241, -42.7006) -> (69.3535, -42.634)
  line L168 (69.3535, -42.634) -> (69.3799, -42.5655)
  line L169 (69.3799, -42.5655) -> (69.4039, -42.4955)
  line L170 (69.4039, -42.4955) -> (69.4257, -42.4241)
  line L171 (69.4257, -42.4241) -> (69.4456, -42.3515)
  line L172 (69.4456, -42.3515) -> (69.4635, -42.2778)
  line L173 (69.4635, -42.2778) -> (69.4796, -42.203)
  line L174 (69.4796, -42.203) -> (69.4941, -42.1273)
  line L175 (69.4941, -42.1273) -> (69.5069, -42.0507)
  line L176 (69.5069, -42.0507) -> (69.5181, -41.9732)
  line L177 (69.5181, -41.9732) -> (69.5278, -41.8949)
  line L178 (69.5278, -41.8949) -> (69.4073, -41.8228)
  line L179 (69.4073, -41.8228) -> (69.2856, -41.7526)
  line L180 (69.2856, -41.7526) -> (69.163, -41.6842)
  line L181 (69.163, -41.6842) -> (69.1, -41.7318)
  line L182 (69.1, -41.7318) -> (69.0385, -41.7802)
  line L183 (69.0385, -41.7802) -> (68.9785, -41.8296)
  line L184 (68.9785, -41.8296) -> (68.9202, -41.88)
  line L185 (68.9202, -41.88) -> (68.8635, -41.9314)
  line L186 (68.8635, -41.9314) -> (68.8086, -41.9838)
  line L187 (68.8086, -41.9838) -> (68.7557, -42.0372)
  line L188 (68.7557, -42.0372) -> (68.7047, -42.0918)
  line L189 (68.7047, -42.0918) -> (68.6561, -42.1476)
  line L190 (68.6561, -42.1476) -> (68.61, -42.2048)
  line L191 (68.61, -42.2048) -> (68.567, -42.2636)
  line L192 (68.567, -42.2636) -> (68.5288, -42.3248)
  line L193 (68.5288, -42.3248) -> (68.3256, -42.7232)
  line L194 (68.3256, -42.7232) -> (68.1363, -42.6297)
  line L195 (68.1363, -42.6297) -> (67.9445, -42.5413)
  line L196 (67.9445, -42.5413) -> (67.7506, -42.458)
  line L197 (67.7506, -42.458) -> (67.5544, -42.3798)
  line L198 (67.5544, -42.3798) -> (67.7146, -41.9622)
  line L199 (67.7146, -41.9622) -> (67.7344, -41.8929)
  line L200 (67.7344, -41.8929) -> (67.7494, -41.8216)
  line L201 (67.7494, -41.8216) -> (67.761, -41.7491)
  line L202 (67.761, -41.7491) -> (67.7699, -41.6756)
  line L203 (67.7699, -41.6756) -> (67.7764, -41.6013)
  line L204 (67.7764, -41.6013) -> (67.7807, -41.5261)
  line L205 (67.7807, -41.5261) -> (67.7829, -41.4503)
  line L206 (67.7829, -41.4503) -> (67.7832, -41.3738)
  line L207 (67.7832, -41.3738) -> (67.7816, -41.2967)
  line L208 (67.7816, -41.2967) -> (67.7782, -41.2191)
  line L209 (67.7782, -41.2191) -> (67.773, -41.141)
  line L210 (67.773, -41.141) -> (67.7662, -41.0623)
  line L211 (67.7662, -41.0623) -> (67.6333, -41.0169)
  line L212 (67.6333, -41.0169) -> (67.4998, -40.9735)
  line L213 (67.4998, -40.9735) -> (67.3656, -40.9322)
  line L214 (67.3656, -40.9322) -> (67.3138, -40.9918)
  line L215 (67.3138, -40.9918) -> (67.2637, -41.052)
  line L216 (67.2637, -41.052) -> (67.2154, -41.1128)
  line L217 (67.2154, -41.1128) -> (67.1688, -41.1742)
  line L218 (67.1688, -41.1742) -> (67.124, -41.2362)
  line L219 (67.124, -41.2362) -> (67.0812, -41.2989)
  line L220 (67.0812, -41.2989) -> (67.0405, -41.3622)
  line L221 (67.0405, -41.3622) -> (67.0021, -41.4261)
  line L222 (67.0021, -41.4261) -> (66.9661, -41.4908)
  line L223 (66.9661, -41.4908) -> (66.9329, -41.5563)
  line L224 (66.9329, -41.5563) -> (66.9031, -41.6227)
  line L225 (66.9031, -41.6227) -> (66.8784, -41.6906)
  line L226 (66.8784, -41.6906) -> (66.7625, -42.1225)
  line L227 (66.7625, -42.1225) -> (66.5579, -42.0705)
  line L228 (66.5579, -42.0705) -> (66.352, -42.0239)
  line L229 (66.352, -42.0239) -> (66.1449, -41.9827)
  line L230 (66.1449, -41.9827) -> (65.9368, -41.947)
  line L231 (65.9368, -41.947) -> (66.0066, -41.5052)
  line L232 (66.0066, -41.5052) -> (66.0116, -41.4333)
  line L233 (66.0116, -41.4333) -> (66.0114, -41.3604)
  line L234 (66.0114, -41.3604) -> (66.0077, -41.2871)
  line L235 (66.0077, -41.2871) -> (66.0012, -41.2134)
  line L236 (66.0012, -41.2134) -> (65.9921, -41.1393)
  line L237 (65.9921, -41.1393) -> (65.9806, -41.0649)
  line L238 (65.9806, -41.0649) -> (65.967, -40.9903)
  line L239 (65.967, -40.9903) -> (65.9514, -40.9154)
  line L240 (65.9514, -40.9154) -> (65.9338, -40.8404)
  line L241 (65.9338, -40.8404) -> (65.9143, -40.7651)
  line L242 (65.9143, -40.7651) -> (65.8931, -40.6898)
  line L243 (65.8931, -40.6898) -> (65.87, -40.6143)
  line L244 (65.87, -40.6143) -> (65.7306, -40.5975)
  line L245 (65.7306, -40.5975) -> (65.5909, -40.5828)
  line L246 (65.5909, -40.5828) -> (65.4511, -40.5702)
  line L247 (65.4511, -40.5702) -> (65.4128, -40.6393)
  line L248 (65.4128, -40.6393) -> (65.3764, -40.7086)
  line L249 (65.3764, -40.7086) -> (65.3417, -40.7781)
  line L250 (65.3417, -40.7781) -> (65.3089, -40.8479)
  line L251 (65.3089, -40.8479) -> (65.278, -40.9179)
  line L252 (65.278, -40.9179) -> (65.2492, -40.988)
  line L253 (65.2492, -40.988) -> (65.2225, -41.0584)
  line L254 (65.2225, -41.0584) -> (65.1982, -41.129)
  line L255 (65.1982, -41.129) -> (65.1765, -41.1998)
  line L256 (65.1765, -41.1998) -> (65.1576, -41.2707)
  line L257 (65.1576, -41.2707) -> (65.1423, -41.3419)
  line L258 (65.1423, -41.3419) -> (65.1322, -41.4133)
  line L259 (65.1322, -41.4133) -> (65.1087, -41.86)
  line L260 (65.1087, -41.86) -> (64.8977, -41.8516)
  line L261 (64.8977, -41.8516) -> (64.6866, -41.8488)
  line L262 (64.6866, -41.8488) -> (64.4755, -41.8516)
  line L263 (64.4755, -41.8516) -> (64.2645, -41.86)
  line L264 (64.2645, -41.86) -> (64.241, -41.4133)
  line L265 (64.241, -41.4133) -> (64.2309, -41.3419)
  line L266 (64.2309, -41.3419) -> (64.2156, -41.2707)
  line L267 (64.2156, -41.2707) -> (64.1967, -41.1998)
  line L268 (64.1967, -41.1998) -> (64.175, -41.129)
  line L269 (64.175, -41.129) -> (64.1506, -41.0584)
  line L270 (64.1506, -41.0584) -> (64.124, -40.988)
  line L271 (64.124, -40.988) -> (64.0952, -40.9179)
  line L272 (64.0952, -40.9179) -> (64.0643, -40.8479)
  line L273 (64.0643, -40.8479) -> (64.0315, -40.7781)
  line L274 (64.0315, -40.7781) -> (63.9968, -40.7086)
  line L275 (63.9968, -40.7086) -> (63.9603, -40.6393)
  line L276 (63.9603, -40.6393) -> (63.9221, -40.5702)
  line L277 (63.9221, -40.5702) -> (63.7822, -40.5828)
  line L278 (63.7822, -40.5828) -> (63.6426, -40.5975)
  line L279 (63.6426, -40.5975) -> (63.5032, -40.6143)
  line L280 (63.5032, -40.6143) -> (63.4801, -40.6898)
  line L281 (63.4801, -40.6898) -> (63.4588, -40.7651)
  line L282 (63.4588, -40.7651) -> (63.4394, -40.8404)
  line L283 (63.4394, -40.8404) -> (63.4218, -40.9154)
  line L284 (63.4218, -40.9154) -> (63.4062, -40.9903)
  line L285 (63.4062, -40.9903) -> (63.3926, -41.0649)
  line L286 (63.3926, -41.0649) -> (63.3811, -41.1393)
  line L287 (63.3811, -41.1393) -> (63.372, -41.2134)
  line L288 (63.372, -41.2134) -> (63.3654, -41.2871)
  line L289 (63.3654, -41.2871) -> (63.3617, -41.3604)
  line L290 (63.3617, -41.3604) -> (63.3615, -41.4333)
  line L291 (63.3615, -41.4333) -> (63.3666, -41.5052)
  line L292 (63.3666, -41.5052) -> (63.4364, -41.947)
  line L293 (63.4364, -41.947) -> (63.2283, -41.9827)
  line L294 (63.2283, -41.9827) -> (63.0212, -42.0239)
  line L295 (63.0212, -42.0239) -> (62.8153, -42.0705)
  line L296 (62.8153, -42.0705) -> (62.6107, -42.1225)
  line L297 (62.6107, -42.1225) -> (62.4948, -41.6906)
  line L298 (62.4948, -41.6906) -> (62.4701, -41.6227)
  line L299 (62.4701, -41.6227) -> (62.4403, -41.5563)
  line L300 (62.4403, -41.5563) -> (62.4071, -41.4908)
  line L301 (62.4071, -41.4908) -> (62.3711, -41.4261)
  line L302 (62.3711, -41.4261) -> (62.3326, -41.3622)
  line L303 (62.3326, -41.3622) -> (62.2919, -41.2989)
  line L304 (62.2919, -41.2989) -> (62.2492, -41.2362)
  line L305 (62.2492, -41.2362) -> (62.2044, -41.1742)
  line L306 (62.2044, -41.1742) -> (62.1578, -41.1128)
  line L307 (62.1578, -41.1128) -> (62.1094, -41.052)
  line L308 (62.1094, -41.052) -> (62.0593, -40.9918)
  line L309 (62.0593, -40.9918) -> (62.0076, -40.9322)
  line L310 (62.0076, -40.9322) -> (61.8734, -40.9735)
  line L311 (61.8734, -40.9735) -> (61.7399, -41.0169)
  line L312 (61.7399, -41.0169) -> (61.607, -41.0623)
  line L313 (61.607, -41.0623) -> (61.6001, -41.141)
  line L314 (61.6001, -41.141) -> (61.595, -41.2191)
  line L315 (61.595, -41.2191) -> (61.5916, -41.2967)
  line L316 (61.5916, -41.2967) -> (61.59, -41.3738)
  line L317 (61.59, -41.3738) -> (61.5903, -41.4503)
  line L318 (61.5903, -41.4503) -> (61.5925, -41.5261)
  line L319 (61.5925, -41.5261) -> (61.5968, -41.6013)
  line L320 (61.5968, -41.6013) -> (61.6032, -41.6756)
  line L321 (61.6032, -41.6756) -> (61.6121, -41.7491)
  line L322 (61.6121, -41.7491) -> (61.6238, -41.8216)
  line L323 (61.6238, -41.8216) -> (61.6387, -41.8929)
  line L324 (61.6387, -41.8929) -> (61.6586, -41.9622)
  line L325 (61.6586, -41.9622) -> (61.8187, -42.3798)
  line L326 (61.8187, -42.3798) -> (61.6226, -42.458)
  line L327 (61.6226, -42.458) -> (61.4286, -42.5413)
  line L328 (61.4286, -42.5413) -> (61.2369, -42.6297)
  line L329 (61.2369, -42.6297) -> (61.0476, -42.7232)
  line L330 (61.0476, -42.7232) -> (60.8444, -42.3248)
  line L331 (60.8444, -42.3248) -> (60.8061, -42.2636)
  line L332 (60.8061, -42.2636) -> (60.7632, -42.2048)
  line L333 (60.7632, -42.2048) -> (60.7171, -42.1476)
  line L334 (60.7171, -42.1476) -> (60.6684, -42.0918)
  line L335 (60.6684, -42.0918) -> (60.6175, -42.0372)
  line L336 (60.6175, -42.0372) -> (60.5645, -41.9838)
  line L337 (60.5645, -41.9838) -> (60.5097, -41.9314)
  line L338 (60.5097, -41.9314) -> (60.453, -41.88)
  line L339 (60.453, -41.88) -> (60.3947, -41.8296)
  line L340 (60.3947, -41.8296) -> (60.3347, -41.7802)
  line L341 (60.3347, -41.7802) -> (60.2732, -41.7318)
  line L342 (60.2732, -41.7318) -> (60.2102, -41.6842)
  line L343 (60.2102, -41.6842) -> (60.0875, -41.7526)
  line L344 (60.0875, -41.7526) -> (59.9659, -41.8228)
  line L345 (59.9659, -41.8228) -> (59.8454, -41.8949)
  line L346 (59.8454, -41.8949) -> (59.855, -41.9732)
  line L347 (59.855, -41.9732) -> (59.8663, -42.0507)
  line L348 (59.8663, -42.0507) -> (59.8791, -42.1273)
  line L349 (59.8791, -42.1273) -> (59.8935, -42.203)
  line L350 (59.8935, -42.203) -> (59.9097, -42.2778)
  line L351 (59.9097, -42.2778) -> (59.9276, -42.3515)
  line L352 (59.9276, -42.3515) -> (59.9474, -42.4241)
  line L353 (59.9474, -42.4241) -> (59.9692, -42.4955)
  line L354 (59.9692, -42.4955) -> (59.9932, -42.5655)
  line L355 (59.9932, -42.5655) -> (60.0197, -42.634)
  line L356 (60.0197, -42.634) -> (60.0491, -42.7006)
  line L357 (60.0491, -42.7006) -> (60.083, -42.7644)
  line L358 (60.083, -42.7644) -> (60.3264, -43.1395)
  line L359 (60.3264, -43.1395) -> (60.1509, -43.2568)
  line L360 (60.1509, -43.2568) -> (59.9784, -43.3786)
  line L361 (59.9784, -43.3786) -> (59.8093, -43.5049)
  line L362 (59.8093, -43.5049) -> (59.6435, -43.6357)
  line L363 (59.6435, -43.6357) -> (59.3619, -43.2882)
  line L364 (59.3619, -43.2882) -> (59.3118, -43.2363)
  line L365 (59.3118, -43.2363) -> (59.2575, -43.1878)
  line L366 (59.2575, -43.1878) -> (59.2006, -43.1414)
  line L367 (59.2006, -43.1414) -> (59.1414, -43.097)
  line L368 (59.1414, -43.097) -> (59.0802, -43.0542)
  line L369 (59.0802, -43.0542) -> (59.0173, -43.0129)
  line L370 (59.0173, -43.0129) -> (58.9527, -42.9731)
  line L371 (58.9527, -42.9731) -> (58.8866, -42.9346)
  line L372 (58.8866, -42.9346) -> (58.8191, -42.8974)
  line L373 (58.8191, -42.8974) -> (58.7502, -42.8616)
  line L374 (58.7502, -42.8616) -> (58.6799, -42.8269)
  line L375 (58.6799, -42.8269) -> (58.6084, -42.7936)
  line L376 (58.6084, -42.7936) -> (58.5026, -42.8859)
  line L377 (58.5026, -42.8859) -> (58.3983, -42.9799)
  line L378 (58.3983, -42.9799) -> (58.2954, -43.0754)
  line L379 (58.2954, -43.0754) -> (58.3211, -43.15)
  line L380 (58.3211, -43.15) -> (58.3482, -43.2235)
  line L381 (58.3482, -43.2235) -> (58.3767, -43.2958)
  line L382 (58.3767, -43.2958) -> (58.4065, -43.3669)
  line L383 (58.4065, -43.3669) -> (58.4379, -43.4366)
  line L384 (58.4379, -43.4366) -> (58.4708, -43.505)
  line L385 (58.4708, -43.505) -> (58.5052, -43.5719)
  line L386 (58.5052, -43.5719) -> (58.5414, -43.6372)